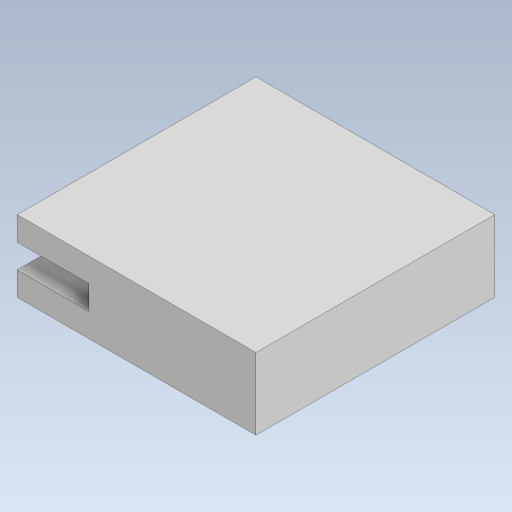
# Autodesk Inventor part: Bracket Lifter Motor
Saved by Autodesk Inventor 2023.5 (Build 275446000, 446)
## iProperties
Created: 2025-09-02
Part Number: Bracket Lifter Motor
Material: Generic
Document SubType Name: Modeling
Designer: Guntur
Density: 1 g/cm^3
Appearance: Default
Author: Guntur
## iProperties of the stored document Bracket Lifter Motor_3DPrint.ipt
Created: 2025-09-02
Part Number: Bracket Lifter Motor_3DPrint
Material: Generic
Document SubType Name: Modeling
Designer: Guntur
Density: 1 g/cm^3
Appearance: Default
Author: Guntur
Autodesk Inventor part; units mm, degrees
ref_plane "YZ Plane" through (0, 0, 0) normal (1, 0, 0) x (0, 1, 0)
ref_plane "XZ Plane" through (0, 0, 0) normal (0, 1, 0) x (-1, 0, 0)
ref_plane "XY Plane" through (0, 0, 0) normal (0, 0, 1) x (1, 0, 0)
sketch "Sketch1" plane through (0, 0, 0) normal (0, 1, 0) x (-1, 0, 0)
  line L0 (10, 10) -> (-10, 10)
  line L1 (-10, 10) -> (-10, -10)
  line L2 (-10, -10) -> (10, -10)
  line L3 (10, -10) -> (10, 10)
  line L4 (10, 10) -> (-10, -10) construction
  line L5 (-10, 10) -> (10, -10) construction
  point P0 (0, 0)
  dimension "d0" = 20
  dimension "d1" = 20
  constraints: 12 end point, 2 midpoint, 2 parallel, 1 horizontal, 1 perpendicular
  measures "d0" distance of L2.end L1.end
  measures "d1" distance of L1.end L0.end
extrude "Extrusion1" add sketch "Sketch1" along normal blind 6
sketch "Sketch2" plane through (-10, 0, 10) normal (0, 0, 1) x (1, 0, 0)
  line L0 (0, 0) -> (0, 6) projected
  line L1 (0, 4) -> (6, 4)
  line L2 (6, 4) -> (6, 2)
  line L3 (6, 2) -> (0, 2)
  line L4 (0, 2) -> (0, 4)
  line L5 (0, 0) -> (20, 0) projected
  point P0 (10, 0)
  point P1 (0, 2)
  dimension "d4" = 6
  dimension "d5" = 2
  dimension "d6" = 2
  constraints: 8 end point, 2 parallel, 1 horizontal, 1 perpendicular, 1 point on line
  measures "d4" distance of L2.end L3.end
  measures "d5" distance of L1.end L2.end
  measures "d6" distance between parallel lines of L3 L5
extrude "Extrusion2" cut sketch "Sketch2" against normal blind 3
sketch "Sketch3" plane through (-10, 0, -10) normal (-1, 0, 0) x (0, 0, 1)
  line L0 (20, 4) -> (17, 4) projected
  line L1 (20, 4) -> (9, 4)
  line L2 (9, 4) -> (9, 2)
  line L3 (9, 2) -> (20, 2)
  line L4 (20, 2) -> (20, 4)
  point P0 (10, 0)
  dimension "d9" = 11
  dimension "d10" = 2
  constraints: 8 end point, 2 parallel, 1 horizontal, 1 perpendicular
  measures "d9" distance of L3.end L2.end
  measures "d10" distance of L2.end L1.end
extrude "Extrusion3" cut sketch "Sketch3" against normal blind 3
body "Solid1"
